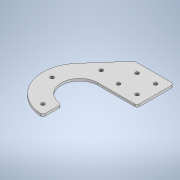
# Autodesk Inventor part: hook v2
Saved by Autodesk Inventor 2022.2 (Build 262287010, 287A)
## iProperties
Created: 2022-01-25
Part Number: hook v2
Material: Generic
Document SubType Name: Modeling
Designer: Robotics
Density: 1 g/cm^3
Appearance: Default
Author: Robotics
Autodesk Inventor part; units mm, degrees
ref_plane "YZ Plane" through (0, 0, 0) normal (1, 0, 0) x (0, 1, 0)
ref_plane "XZ Plane" through (0, 0, 0) normal (0, 1, 0) x (-1, 0, 0)
ref_plane "XY Plane" through (0, 0, 0) normal (0, 0, 1) x (1, 0, 0)
sketch "Sketch3" plane through (0, 0, 0) normal (0, 1, 0) x (-1, 0, 0)
  arc A0 (0, 0) -> (-0.5498, 50.794) centre (-0.5498, 25.394) ccw
  arc A1 (37.5561, -8.2003) -> (-0.5498, 76.194) centre (-0.5498, 25.394) ccw
  line L0 (0, 0) -> (-53.975, 0)
  line L1 (-53.975, 0) -> (-53.975, -50.8)
  line L2 (-53.975, -50.8) -> (0, -50.8)
  line L3 (0, -50.8) -> (37.5561, -8.2003)
  line L4 (-0.5498, 76.194) -> (-0.5498, 50.794)
  line L5 (50.2502, 25.394) -> (37.5502, 25.394)
  circle A2 centre (37.5502, 25.394) radius 2.3812
  line L6 (24.8487, 25.6689) -> (12.1517, 25.394)
  line L7 (12.1517, 25.394) -> (12.1517, 85.7885)
  line L8 (12.1517, 85.7885) -> (12.1517, 25.394)
  line L9 (12.1517, 25.394) -> (12.1517, -39.1077)
  line L10 (-0.5498, 63.494) -> (12.1517, 63.494)
  line L11 (12.1517, 3.3979) -> (12.1517, -37.0164)
  line L12 (12.1517, -16.8093) -> (14.0122, -16.8093)
  circle A3 centre (12.1517, -16.8093) radius 2.3812
  circle A4 centre (12.1517, 63.494) radius 2.3812
  dimension "d19" = 25.4
  dimension "d20" = 25.4
  dimension "d21" = 53.975
  dimension "d22" = 50.8
  dimension "d23" = 53.975
  dimension "d39" = 12.7
  dimension "d40" = 4.7625
  dimension "d42" = 12.7
  dimension "d43" = 4.7625
  dimension "d44" = 4.7625
  constraints: 26 end point, 7 point on circle, 6 point on line, 5 centre point, 3 coincident, 3 horizontal, 3 perpendicular, 2 midpoint, 2 vertical, 1 collinear, 1 tangent
  measures "d19" radius of A0
  measures "d20" radial gap between concentric circles of A0 A1
  measures "d21" distance of L0.start L0.end
  measures "d22" distance of L0.end L1.end
  measures "d23" distance of L1.end L2.end
  measures "d39" distance of L5.start L5.end
  measures "d40" diameter of A2
  measures "d42" distance of L6.start L6.end
  measures "d43" diameter of A3
  measures "d44" diameter of A4
extrude "Extrusion3" add sketch "Sketch3" along normal blind 3.175 contours A0 L9 A3 L3 L2 L1 L0 | A2 | A0 L7 A4 A1 L3 L9 A3 | A3 L9 | L9 A3 | A0 L4 L10 A4 L7 | A4 L10 L7 | L7 A4 | L4 A1 L7 A4 L10 | L10 A4 L7
fillet "Fillet3" radius 3.175 5 edges at (0, 1.5875, -50.8) (53.975, 1.5875, -50.8) (53.975, 1.5875, 0) (0.5498, 1.5875, 50.794) (0.5498, 1.5875, 76.194)
sketch "Sketch4" plane through (0, 3.175, 0) normal (0, 1, 0) x (1, 0, 0)
  line L0 (53.975, 3.175) -> (53.975, 47.625) projected
  line L1 (53.975, 25.4) -> (41.275, 25.4)
  line L2 (41.275, 25.4) -> (41.275, 38.1)
  line L3 (41.275, 38.1) -> (41.275, 12.7)
  line L4 (41.275, 12.7) -> (15.875, 12.7)
  point P0 (0, 0)
  point P1 (15.875, 38.1)
  dimension "d27" = 12.7
  dimension "d28" = 12.7
  dimension "d29" = 25.4
  dimension "d30" = 25.4
  dimension "d31" = 25.4
  constraints: 8 end point, 2 perpendicular, 1 horizontal, 1 midpoint, 1 point on line
  measures "d27" distance of L1.start L1.end
  measures "d28" distance of L1.end L2.end
  measures "d29" distance of L2.end L3.end
  measures "d30" distance of L3.end L4.end
  measures "d31" distance of L4.end point (15.875, 38.1)
hole "Hole1" at (15.875, 3.175, -38.1) at (15.875, 3.175, -12.7) at (41.275, 3.175, -12.7) at (41.275, 3.175, -38.1) direction (0, -1, 0) diameter 4.7625 end through all
extrude "Extrusion4" cut sketch "Sketch3" along normal blind 3.175 contours A2 | A3 L9 | L9 A3 | A4 L10 L7 | L7 A4 | L10 A4 L7
body "Solid2"
